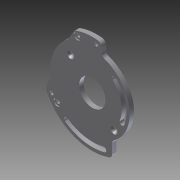
# Autodesk Inventor part: motor plate
Saved by Autodesk Inventor 2012 (Build 160160000, 160)
## iProperties
Created: 2012-01-30
Part Number: motor plate
Material: Default
Document SubType Name: Modeling
Designer: Antonella Wilby
Density: 1 g/cm^3
Mass: 66.7575 g
Surface Area: 265.079 cm^2
Volume: 66.7575 cm^3
Author: Antonella Wilby
Autodesk Inventor part; units mm, degrees
ref_plane "YZ Plane" through (0, 0, 0) normal (1, 0, 0) x (0, 1, 0)
ref_plane "XZ Plane" through (0, 0, 0) normal (0, 1, 0) x (-1, 0, 0)
ref_plane "XY Plane" through (0, 0, 0) normal (0, 0, 1) x (1, 0, 0)
sketch "Sketch1" plane through (0, 0, 0) normal (0, 0, 1) x (1, 0, 0)
  circle A0 centre (0, 0) radius 53.975 construction
  circle A1 centre (0, 0) radius 19.05
  line L0 (-100.2597, 0) -> (86.9261, 0) projected
  line L1 (0, -117.8456) -> (0, 102.763) projected
  line L2 (13.4938, 63.0969) -> (13.4937, 56.9678)
  arc A2 (-66.1831, -30.8617) -> (24.3417, -68.8486) centre (0, 0) ccw
  arc A3 (7.8581, 69.4066) -> (-23.8901, 65.6375) centre (0, 0) ccw
  arc A4 (31.2487, -44.0093) -> (17.7549, 50.9712) centre (0, 0) ccw
  arc A5 (13.4937, 56.9678) -> (17.7549, 50.9712) centre (19.8438, 56.9678) ccw
  arc A6 (13.4938, 63.0969) -> (7.8581, 69.4066) centre (7.1437, 63.0969) ccw
  line L3 (28.575, -49.1869) -> (28.575, -62.8618)
  arc A7 (24.3417, -68.8486) -> (28.575, -62.8618) centre (22.225, -62.8618) ccw
  arc A8 (31.2487, -44.0093) -> (28.575, -49.1869) centre (34.925, -49.1869) ccw
  line L4 (-61.0828, -12.5629) -> (-66.1138, -22.8801)
  arc A9 (-66.1138, -22.8801) -> (-66.1831, -30.8617) centre (-57.7807, -26.9436) ccw
  line L5 (0, 0) -> (-57.7807, -26.9436) construction
  arc A10 (-36.5638, 47.9812) -> (-59.9899, -6.35) centre (0, 0) ccw
  arc A11 (-61.0828, -12.5629) -> (-59.9899, -6.35) centre (-71.3564, -7.5532) ccw
  line L6 (-34.9493, 49.7953) -> (-27.1815, 62.9071)
  arc A12 (-36.5638, 47.9812) -> (-34.9493, 49.7953) centre (-40.4126, 53.0319) ccw
  arc A13 (-23.8901, 65.6375) -> (-27.1815, 62.9071) centre (-21.7183, 59.6705) ccw
  line L7 (0, 0) -> (-21.7183, 59.6705) construction
  point P0 (13.4937, 68.5342)
  point P1 (28.575, -45.7905)
  point P2 (28.575, -67.2021)
  point P3 (-67.9722, -26.6913)
  point P4 (-53.975, 0)
  dimension "d0" = 107.95
  dimension "d10" = 38.1
  dimension "d48" = 6.35
  dimension "d58" = 6.35
  dimension "d59" = 28.575
  dimension "d60" = 73.025
  dimension "d75" = 65
  dimension "d86" = 60.325
  dimension "d88" = 6.35
  dimension "d91" = 6.35
  dimension "d92" = 69.85
  dimension "d119" = 11.43
  dimension "d120" = 9.271
  dimension "d123" = 13.4938
  dimension "d124" = 20
  dimension "d126" = 15.24
  constraints: 28 point on circle, 16 tangent, 13 centre point, 12 end point, 5 point on line, 4 coincident, 3 equal radius, 1 horizontal alignment, 1 parallel, 4 other
  measures "d10" diameter of A1
  measures "d48" radius of A5
  measures "d58" radius of A7
  measures "d59" distance between parallel lines of L1 L3
  measures "d60" radius of A2
  measures "d75" angle of L5 L1
  measures "d86" radius of A10
  measures "d88" distance from line of L0 A10.end
  measures "d91" radius of A12
  measures "d92" radius of A3
  measures "d119" radius of A11
  measures "d120" radius of A9
  measures "d123" distance between parallel lines of L1 L2
  measures "d124" angle of L1 L7
  measures "d126" distance of L6.start L6.end
extrude "Base" add sketch "Sketch1" along normal mid plane 6.35 contours L0 A4 A8 L3 A7 A2 L1 A1 | A1 L1 A3 A6 L2 A5 A4 L0 | A1 L0 A10 A12 L6 A13 A3 L1 | L1 A2 A9 L4 A11 A10 L0 A1
sketch "Sketch5" plane through (0, 0, 3.175) normal (0, 0, 1) x (1, 0, 0)
  circle A0 centre (0, 0) radius 19.05 projected
  arc A1 (31.2487, -44.0093) -> (17.7549, 50.9712) centre (0, 0) ccw projected
  line L0 (-100.2597, 0) -> (86.9261, 0) projected
  line L1 (0, -117.5661) -> (0, 101.086) projected
  line L2 (0, 0) -> (-31.4309, 31.4309) construction
  arc A2 (-66.1831, -30.8617) -> (24.3417, -68.8486) centre (0, 0) ccw projected
  line L3 (31.4309, -31.4309) -> (0, 0) construction
  dimension "d49" = 45
  dimension "d50" = 44.45
  dimension "d109" = 44.45
  constraints: 4 end point, 1 collinear
  measures "d49" angle of L1 L2
  measures "d50" distance of A0.centre L2.end
  measures "d109" distance of L3.start L3.end
hole "Motor Mount Hole" at (-31.4309, 31.4309, 3.175) at (31.4309, -31.4309, 3.175) direction (0, 0, -1) diameter 5.1054 end through all countersink diameter 9.779 countersink angle 82 clearance for "Flat Head Machine Screw (82)" size "#10" standard "Ansi Unified Screw Threads"
sketch "Sketch6" plane through (0, 0, 3.175) normal (0, 0, 1) x (1, 0, 0)
  arc A0 (-66.1831, -30.8617) -> (24.3417, -68.8486) centre (0, 0) ccw projected
  line L0 (-99.0177, 0) -> (79.4738, 0) projected
  line L1 (0, -117.5661) -> (0, 101.086) projected
  line L2 (0, 0) -> (-21.7183, 59.6705) construction
  arc A1 (-36.5638, 47.9812) -> (-59.9899, -6.35) centre (0, 0) ccw projected
  line L3 (-51.0449, -37.7712) -> (0, 0) construction
  dimension "d114" = 63.5
  dimension "d121" = 63.5
  dimension "d122" = 53.5
  dimension "d127" = 20
  constraints: 4 end point
  measures "d114" distance of L2.start L2.end
  measures "d121" distance of L3.start L3.end
  measures "d122" angle of L1 L3
  measures "d127" angle of L1 L2
hole "Standoffs holes to front plate" at (-51.0449, -37.7712, 3.175) at (-21.7183, 59.6705, 3.175) direction (0, 0, -1) diameter 5.1054 end through all counterbore diameter 9.779 counterbore depth 1.5875 clearance for "Flat Head Machine Screw (82)" size "#10" standard "Ansi Unified Screw Threads"
sketch "Sketch8" plane through (0, 0, -3.175) normal (0, 0, -1) x (-1, 0, 0)
  arc A0 (23.8901, 65.6375) -> (-7.8581, 69.4066) centre (0, 0) ccw projected
  line L0 (91.3248, 0) -> (-78.1916, 0) projected
  line L1 (0, -101.8795) -> (0, 100.1019) projected
  line L2 (0, 0) -> (-5.5344, 63.2584) construction
  arc A1 (59.9899, -6.35) -> (36.5638, 47.9812) centre (0, 0) ccw projected
  line L3 (0, 0) -> (58.7006, -29.9095) construction
  point P0 (54.0079, -0.6455)
  dimension "d103" = 63.5
  dimension "d104" = 5
  dimension "d110" = 27
  dimension "d111" = 65.8812
  constraints: 4 end point
  measures "d103" distance of L2.start L2.end
  measures "d104" angle of L1 L2
  measures "d110" angle of L0 L3
  measures "d111" distance of L3.start L3.end
hole "Standoff holes to back plate" at (-58.7006, -29.9095, -3.175) at (5.5344, 63.2584, -3.175) direction (0, 0, 1) diameter 5.1054 end through all counterbore diameter 9.779 counterbore depth 1.5875 clearance for "Flat Head Machine Screw (82)" size "#10" standard "Ansi Unified Screw Threads"
sketch "Sketch7" plane through (0, 0, 3.175) normal (0, 0, 1) x (1, 0, 0)
  arc A0 (-66.1831, -30.8617) -> (24.3417, -68.8486) centre (0, 0) ccw projected
  arc A1 (31.2487, -44.0093) -> (17.7549, 50.9712) centre (0, 0) ccw projected
  arc A2 (-35.2784, -50.3828) -> (-39.1538, -55.9174) centre (-37.2161, -53.1501) ccw
  arc A3 (17.6676, -65.9365) -> (15.919, -59.4103) centre (16.7933, -62.6734) ccw
  arc A4 (-35.2784, -50.3828) -> (15.919, -59.4103) centre (0, 0) ccw
  arc A5 (-39.1538, -55.9174) -> (17.6676, -65.9365) centre (0, 0) ccw
  line L0 (-100.2597, 0) -> (86.9261, 0) projected
  line L1 (0, -117.5661) -> (0, 101.086) projected
  line L2 (16.7933, -62.6734) -> (0, 0) construction
  line L3 (0, 0) -> (-37.2161, -53.1501) construction
  dimension "d69" = 4.7625
  dimension "d70" = 6.7564
  dimension "d71" = 75
  dimension "d72" = 55
  constraints: 14 point on circle, 4 centre point, 4 end point, 4 tangent
  measures "d69" radial gap between concentric circles of A5 A0
  measures "d70" radial gap between concentric circles of A4 A5
  measures "d71" angle of L0 L2
  measures "d72" angle of L0 L3
extrude "Tensioning Slot" cut sketch "Sketch7" against normal through all
sketch "Sketch10" plane through (0, 0, 3.175) normal (0, 0, 1) x (1, 0, 0)
  arc A0 (31.2487, -44.0093) -> (17.7549, 50.9712) centre (0, 0) ccw projected
  arc A1 (-66.1831, -30.8617) -> (24.3417, -68.8486) centre (0, 0) ccw projected
  line L0 (-100.2597, 0) -> (86.9261, 0) projected
  line L1 (0, -117.5661) -> (0, 101.086) projected
  arc A2 (34.3327, 35.2581) -> (29.6192, 30.4175) centre (31.9759, 32.8378) ccw
  arc A3 (39.6072, -15.2903) -> (45.9102, -17.7236) centre (42.7587, -16.507) ccw
  line L2 (0, 0) -> (31.9759, 32.8378) construction
  arc A4 (45.9102, -17.7236) -> (34.3327, 35.2581) centre (0, 0) ccw
  arc A5 (39.6072, -15.2903) -> (29.6192, 30.4175) centre (0, 0) ccw
  line L3 (42.7587, -16.507) -> (0, 0) construction
  dimension "d130" = 4.7625
  dimension "d131" = 6.7564
  constraints: 12 point on circle, 4 centre point, 4 end point, 3 tangent, 2 point on line
  measures "d130" radial gap between concentric circles of A0 A4
  measures "d131" radial gap between concentric circles of A5 A4
extrude "Extrusion3" cut sketch "Sketch10" against normal through all
body "Solid1"
